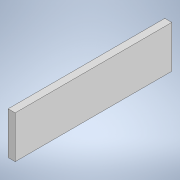
# Autodesk Inventor part: pinho 25x150
Saved by Autodesk Inventor 2020 (Build 240168000, 168)
## iProperties
Created: 2021-05-15
Part Number: pinho 25x150
Material: Generic
Document SubType Name: Modeling
Designer: super
Density: 1 g/cm^3
Appearance: Default
Author: super
Autodesk Inventor part; units mm, degrees
ref_plane "YZ Plane" through (0, 0, 0) normal (1, 0, 0) x (0, 1, 0)
ref_plane "XZ Plane" through (0, 0, 0) normal (0, 1, 0) x (-1, 0, 0)
ref_plane "Work Plane1" through (0, -551.3204, 0) normal (0, 0, -1) x (1, 0, 0)
sketch "Sketch1" plane through (0, -551.3204, 0) normal (0, 0, -1) x (1, 0, 0)
  line L0 (0, -350.6602) -> (25, -350.6602)
  line L1 (25, -350.6602) -> (25, -200.6602)
  line L2 (25, -200.6602) -> (0, -200.6602)
  line L3 (0, -200.6602) -> (0, -350.6602)
  point P0 (0, -551.3204)
  dimension "d0" = 25
  dimension "d1" = 150
  constraints: 8 end point, 2 parallel, 1 horizontal, 1 perpendicular
  measures "d0" distance of L2.end L1.end
  measures "d1" distance of L1.end L0.end
extrude "Extrusion1" add sketch "Sketch1" along normal blind 556
body "Solid1"
